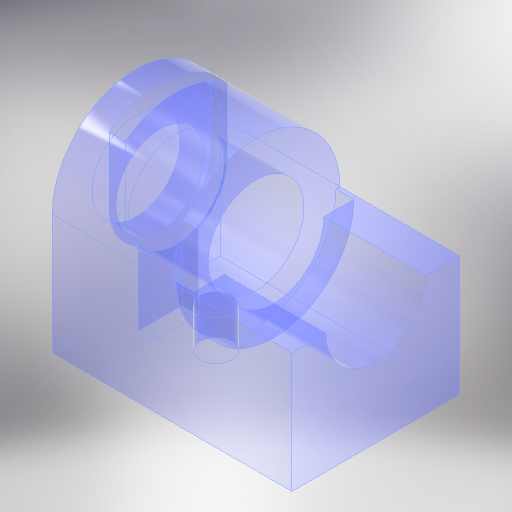
# Autodesk Inventor part: raman-colimeter-holder
Saved by Autodesk Inventor 2026 (Build 300175050, 175E)
## iProperties
Created: 2025-10-28
Part Number: raman-colimeter-holder
Material: ABS プラスチック
Document SubType Name: Modeling
Designer: jin20
Density: 1.06 g/cm^3
Appearance: クリア - 青
Author: jin20
Autodesk Inventor part; units mm, degrees
ref_plane "YZ Plane" through (0, 0, 0) normal (1, 0, 0) x (0, 1, 0)
ref_plane "XZ Plane" through (0, 0, 0) normal (0, 1, 0) x (-1, 0, 0)
ref_plane "XY Plane" through (0, 0, 0) normal (0, 0, 1) x (1, 0, 0)
sketch "スケッチ1" plane through (0, 0, 0) normal (1, 0, 0) x (0, 1, 0)
  line L0 (-30, 0) -> (-30, 21)
  line L1 (-30, 21) -> (0, 21)
  line L2 (0, 21) -> (0, 0)
  line L3 (-30, 0) -> (-30, -21)
  line L4 (-30, -21) -> (0, -21)
  line L5 (0, -21) -> (0, 0)
  arc A0 (0, -21) -> (0, 21) centre (0, 0) ccw
  dimension "d0" = 30
  dimension "d1" = 21
  constraints: 12 end point, 2 point on circle, 1 centre point, 1 coincident, 1 parallel
  measures "d0" distance of L0.end L1.end
  measures "d1" distance of L0.start L0.end
extrude "押し出し1" add sketch "スケッチ1" along normal mid plane 60
sketch "スケッチ2" plane through (30, 0, 0) normal (1, 0, 0) x (0, 0, -1)
  arc A0 (-12.5, 0) -> (12.5, 0) centre (0, 0) ccw
  arc A1 (21, 0) -> (-21, 0) centre (0, 0) ccw
  line L0 (-21, 0) -> (-12.5, 0)
  line L1 (12.5, 0) -> (21, 0)
  dimension "d4" = 25
  constraints: 4 end point, 4 point on circle, 2 centre point, 2 coincident
  measures "d4" diameter of A0
extrude "押し出し2" cut sketch "スケッチ2" against normal blind 30
sketch "スケッチ3" plane through (0, 0, 0) normal (0, 1, 0) x (-1, 0, 0)
  line L0 (0, 0) -> (-4.5, 0)
  line L1 (-4.5, 0) -> (-4.5, 20)
  line L2 (-4.5, 20) -> (0, 20)
  line L3 (0, 20) -> (0, 0)
  line L4 (42, 0) -> (-42, 0) projected
  dimension "d7" = 4.5
  dimension "d8" = 20
  constraints: 8 end point, 2 parallel, 1 horizontal, 1 perpendicular
  measures "d7" distance of L1.end L2.end
  measures "d8" distance of L0.end L1.end
revolve "回転1" cut sketch "スケッチ3" angle 360 about axis through (-10, 0, 0) along (1, 0, 0)
sketch "スケッチ4" plane through (0, 0, 0) normal (1, 0, 0) x (0, 0, -1)
  circle A0 centre (0, 0) radius 12
  dimension "d15" = 24
  constraints: 1 centre point, 1 coincident
  measures "d15" diameter of A0
extrude "押し出し3" cut sketch "スケッチ4" against normal blind 20
sketch "スケッチ6" plane through (0, 0, 0) normal (0, 1, 0) x (-1, 0, 0)
  line L0 (20, -12) -> (20, 12) projected
  line L1 (20, 0) -> (24, 0)
  line L2 (24, 0) -> (24, 12.75)
  line L3 (24, 12.75) -> (20, 12.75)
  line L4 (20, 12.75) -> (20, 0)
  line L5 (42, 0) -> (-42, 0) projected
  point P0 (0, 0)
  dimension "d16" = 4
  dimension "d17" = 12.75
  constraints: 8 end point, 2 parallel, 1 horizontal, 1 midpoint, 1 perpendicular
  measures "d16" distance of L3.end L2.end
  measures "d17" distance of L2.end L1.end
revolve "回転3" cut sketch "スケッチ6" angle 360 about axis through (-10, 0, 0) along (1, 0, 0)
sketch "スケッチ7" plane through (-30, 0, 0) normal (-1, 0, 0) x (0, 0, 1)
  circle A0 centre (0, 0) radius 11
  dimension "d19" = 22
  constraints: 1 centre point, 1 coincident
  measures "d19" diameter of A0
extrude "押し出し4" cut sketch "スケッチ7" against normal through all
sketch "スケッチ8" plane through (0, 0, 0) normal (0, 1, 0) x (-1, 0, 0)
  line L0 (20, 12.75) -> (24, 12.75) projected
  line L1 (24, 0) -> (24, 12.75)
  line L2 (24, 12.75) -> (20, 12.75)
  line L3 (20, 12.75) -> (20, 0)
  line L4 (20, -12.75) -> (24, -12.75)
  line L5 (24, 0) -> (24, -12.75)
  line L6 (20, -12.75) -> (20, 0)
  point P0 (0, 0)
  constraints: 12 end point, 2 point on line, 1 parallel
extrude "押し出し5" cut sketch "スケッチ8" along normal through all
sketch "スケッチ9" plane through (0, 0, 0) normal (0, 1, 0) x (-1, 0, 0)
  line L0 (24, 0) -> (24, -5.5)
  line L1 (24, -5.5) -> (20, -5.5)
  line L2 (20, -5.5) -> (20, 0)
  line L3 (24, 0) -> (24, 5.5)
  line L4 (24, 5.5) -> (20, 5.5)
  line L5 (20, 5.5) -> (20, 0)
  point P0 (0, 0)
  dimension "d24" = 4
  dimension "d25" = 5.5
  constraints: 12 end point, 1 parallel
  measures "d24" distance of L0.end L1.end
  measures "d25" distance of L0.start L0.end
extrude "押し出し6" cut sketch "スケッチ9" against normal through all
sketch "スケッチ10" plane through (-30, -30, -21) normal (0, -1, 0) x (1, 0, 0)
  line L0 (30, 21) -> (20, 21) construction
  circle A0 centre (20, 21) radius 4
  dimension "d28" = 10
  dimension "d29" = 8
  constraints: 2 end point, 1 centre point, 1 coincident, 1 horizontal
  measures "d28" distance of L0.start L0.end
  measures "d29" diameter of A0
extrude "押し出し7" cut sketch "スケッチ10" against normal blind 10
